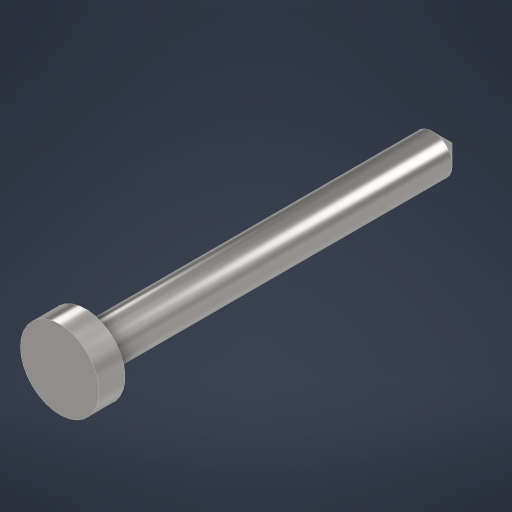
# Autodesk Inventor part: Langbektang houder
Saved by Autodesk Inventor 2023.2 (Build 272271000, 271)
## iProperties
Created: 2020-09-09
Part Number: Langbektang houder
Material: Steel, Mild
Document SubType Name: Modeling
Designer: nathan.bollaert
Density: 7.85 g/cm^3
Appearance: Semi-Polished
Author: nathan.bollaert
Autodesk Inventor part; units mm, degrees
ref_plane "YZ Plane" through (0, 0, 0) normal (1, 0, 0) x (0, 1, 0)
ref_plane "XZ Plane" through (0, 0, 0) normal (0, 1, 0) x (-1, 0, 0)
ref_plane "XY Plane" through (0, 0, 0) normal (0, 0, 1) x (1, 0, 0)
sketch "Sketch1" plane through (0, 0, 0) normal (0, 1, 0) x (-1, 0, 0)
  line L0 (0, 0) -> (0, -15)
  line L1 (0.75, -1) -> (1.5, -1)
  line L2 (1.5, -1) -> (1.5, 0)
  line L3 (1.5, 0) -> (0, 0)
  line L4 (0, -15) -> (0.75, -14.25)
  line L5 (0.75, -1) -> (0.75, -14.25)
  dimension "d230" = 1
  dimension "d231" = 3
  dimension "d232" = 45
  dimension "d233" = 14
  dimension "d234" = 1.5
  constraints: 12 end point, 3 perpendicular, 2 vertical, 1 point on line
  measures "d230" distance of L1.end L2.end
  measures "d231" diameter of L2.end L0
  measures "d232" angle of L0 L4
  measures "d233" distance from line of L0.end L1
  measures "d234" diameter of L5 L0
revolve "Revolution1" add sketch "Sketch1" angle 360 about axis through (0, 0, 0) along (0, 0, -1)
body "Solid5"
